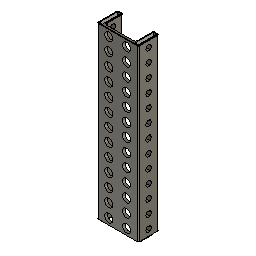
nxp_s32g3_support_plate (Autodesk Fusion 360 archive; units mm, degrees)
design "2u(ish) rail"
Autodesk Fusion 360 part; units mm, degrees
sketch "Sketch1" plane through (0, 0, 0) normal (0, 1, 0) x (1, 0, 0)
  line L0 (0, 0) -> (31.75, 0)
  line L1 (31.75, 0) -> (31.75, -130.8125)
  line L2 (31.75, -130.8125) -> (0, -130.8125)
  line L3 (0, -130.8125) -> (0, 0)
  line L4 (0, 0) -> (4.25, 0)
  line L5 (31.75, 0) -> (27.5, 0)
  line L6 (27.5, 0) -> (27.5, -130.8125)
  line L7 (4.25, 0) -> (4.25, -130.8125)
  circle A0 centre (9.0625, -5.0313) radius 3.1
  circle A1 centre (22.6875, -5.0313) radius 3.1
  circle A2 centre (9.0625, -15.0938) radius 3.1
  circle A3 centre (22.6875, -15.0938) radius 3.1
  circle A4 centre (9.0625, -25.1563) radius 3.1
  circle A5 centre (22.6875, -25.1563) radius 3.1
  circle A6 centre (9.0625, -35.2188) radius 3.1
  circle A7 centre (22.6875, -35.2188) radius 3.1
  circle A8 centre (9.0625, -45.2813) radius 3.1
  circle A9 centre (22.6875, -45.2813) radius 3.1
  circle A10 centre (9.0625, -55.3438) radius 3.1
  circle A11 centre (22.6875, -55.3438) radius 3.1
  circle A12 centre (9.0625, -65.4063) radius 3.1
  circle A13 centre (22.6875, -65.4063) radius 3.1
  circle A14 centre (9.0625, -75.4688) radius 3.1
  circle A15 centre (22.6875, -75.4688) radius 3.1
  circle A16 centre (9.0625, -85.5313) radius 3.1
  circle A17 centre (22.6875, -85.5313) radius 3.1
  circle A18 centre (9.0625, -95.5938) radius 3.1
  circle A19 centre (22.6875, -95.5938) radius 3.1
  circle A20 centre (9.0625, -105.6563) radius 3.1
  circle A21 centre (22.6875, -105.6563) radius 3.1
  circle A22 centre (9.0625, -115.7188) radius 3.1
  circle A23 centre (22.6875, -115.7188) radius 3.1
  circle A24 centre (9.0625, -125.7813) radius 3.1
  circle A25 centre (22.6875, -125.7813) radius 3.1
  dimension "d8" = 31.75
  dimension "d9" = 130.8125
  dimension "d11" = 4.25
  dimension "d12" = 4.25
  dimension "d15" = 6.2
  dimension "d16" = 5.0313
  dimension "d17" = 9.0625
  dimension "d18" = 6.2
  dimension "d19" = 5.0313
  dimension "d20" = 9.0625
  dimension "d23" = 10.0625
  dimension "d24" = 0
  constraint horizontal L0
  constraint vertical L1
  constraint horizontal L2
  constraint vertical L3
  constraint coincident L0.start L3.end
  constraint coincident L0 L4.end
  constraint perpendicular L1 L5
  constraint coincident L2 L6.end
  constraint perpendicular L2 L6
  constraint coincident L2 L7.end
  constraint perpendicular L2 L7
  measures "d8" distance of L0.start L0.end
  measures "d9" distance of L0.start L2.end
  measures "d11" distance of L0.start L4.end
  measures "d12" distance of L1 L6
  measures "d15" diameter of A0
  measures "d16" distance of L0 A0.centre
  measures "d17" distance of L3 A0.centre
  measures "d18" diameter of A1
  measures "d19" distance of L0 A1.centre
  measures "d20" distance of L1 A1.centre
extrude "Extrude1" add sketch "Sketch1" along normal blind 2 contours L0 L2 L6 L7 makes body 1
sketch "Sketch2" plane through (0, 0, 0) normal (0, 1, 0) x (1, 0, 0)
extrude "Extrude2" add sketch "Sketch1" along normal blind 15.875 contours L0 L2 L3 L4 L7 | L0 L1 L2 L5 L6 bodies 1
sketch "Sketch3" plane through (31.75, 0, 0) normal (1, 0, 0) x (0, 1, 0)
  line L0 (0, 130.8125) -> (0, 0)
  line L1 (0, 0) -> (15.875, 0)
  line L2 (15.875, 0) -> (15.875, 130.8125)
  line L3 (15.875, 130.8125) -> (0, 130.8125)
  circle A0 centre (7.9375, 5.0313) radius 2
  line L4 (0, 0) -> (0, 130.8125)
  line L5 (9.0922, 3.0313) -> (10.2469, 5.0313)
  line L6 (10.2469, 5.0313) -> (9.0922, 7.0313)
  line L7 (9.0922, 7.0313) -> (6.7828, 7.0313)
  line L8 (6.7828, 7.0313) -> (5.6281, 5.0313)
  line L9 (5.6281, 5.0313) -> (6.7828, 3.0313)
  line L10 (6.7828, 3.0313) -> (9.0922, 3.0313)
  line L11 (10.2469, 15.0938) -> (9.0922, 17.0938)
  line L12 (9.0922, 13.0938) -> (10.2469, 15.0938)
  line L13 (6.7828, 13.0938) -> (9.0922, 13.0938)
  line L14 (5.6281, 15.0938) -> (6.7828, 13.0938)
  line L15 (6.7828, 17.0938) -> (5.6281, 15.0938)
  line L16 (9.0922, 17.0938) -> (6.7828, 17.0938)
  line L17 (10.2469, 25.1563) -> (9.0922, 27.1563)
  line L18 (9.0922, 23.1563) -> (10.2469, 25.1563)
  line L19 (6.7828, 23.1563) -> (9.0922, 23.1563)
  line L20 (5.6281, 25.1563) -> (6.7828, 23.1563)
  line L21 (6.7828, 27.1563) -> (5.6281, 25.1563)
  line L22 (9.0922, 27.1563) -> (6.7828, 27.1563)
  line L23 (10.2469, 35.2188) -> (9.0922, 37.2188)
  line L24 (9.0922, 33.2188) -> (10.2469, 35.2188)
  line L25 (6.7828, 33.2188) -> (9.0922, 33.2188)
  line L26 (5.6281, 35.2188) -> (6.7828, 33.2188)
  line L27 (6.7828, 37.2188) -> (5.6281, 35.2188)
  line L28 (9.0922, 37.2188) -> (6.7828, 37.2188)
  line L29 (10.2469, 45.2813) -> (9.0922, 47.2813)
  line L30 (9.0922, 43.2813) -> (10.2469, 45.2813)
  line L31 (6.7828, 43.2813) -> (9.0922, 43.2813)
  line L32 (5.6281, 45.2813) -> (6.7828, 43.2813)
  line L33 (6.7828, 47.2813) -> (5.6281, 45.2813)
  line L34 (9.0922, 47.2813) -> (6.7828, 47.2813)
  line L35 (10.2469, 55.3438) -> (9.0922, 57.3438)
  line L36 (9.0922, 53.3438) -> (10.2469, 55.3438)
  line L37 (6.7828, 53.3438) -> (9.0922, 53.3438)
  line L38 (5.6281, 55.3438) -> (6.7828, 53.3438)
  line L39 (6.7828, 57.3438) -> (5.6281, 55.3438)
  line L40 (9.0922, 57.3438) -> (6.7828, 57.3438)
  line L41 (10.2469, 65.4063) -> (9.0922, 67.4063)
  line L42 (9.0922, 63.4063) -> (10.2469, 65.4063)
  line L43 (6.7828, 63.4063) -> (9.0922, 63.4063)
  line L44 (5.6281, 65.4063) -> (6.7828, 63.4063)
  line L45 (6.7828, 67.4063) -> (5.6281, 65.4063)
  line L46 (9.0922, 67.4063) -> (6.7828, 67.4063)
  line L47 (10.2469, 75.4688) -> (9.0922, 77.4688)
  line L48 (9.0922, 73.4688) -> (10.2469, 75.4688)
  line L49 (6.7828, 73.4688) -> (9.0922, 73.4688)
  line L50 (5.6281, 75.4688) -> (6.7828, 73.4688)
  line L51 (6.7828, 77.4688) -> (5.6281, 75.4688)
  line L52 (9.0922, 77.4688) -> (6.7828, 77.4688)
  line L53 (10.2469, 85.5313) -> (9.0922, 87.5313)
  line L54 (9.0922, 83.5313) -> (10.2469, 85.5313)
  line L55 (6.7828, 83.5313) -> (9.0922, 83.5313)
  line L56 (5.6281, 85.5313) -> (6.7828, 83.5313)
  line L57 (6.7828, 87.5313) -> (5.6281, 85.5313)
  line L58 (9.0922, 87.5313) -> (6.7828, 87.5313)
  line L59 (10.2469, 95.5938) -> (9.0922, 97.5938)
  line L60 (9.0922, 93.5938) -> (10.2469, 95.5938)
  line L61 (6.7828, 93.5938) -> (9.0922, 93.5938)
  line L62 (5.6281, 95.5938) -> (6.7828, 93.5938)
  line L63 (6.7828, 97.5938) -> (5.6281, 95.5938)
  line L64 (9.0922, 97.5938) -> (6.7828, 97.5938)
  line L65 (10.2469, 105.6563) -> (9.0922, 107.6563)
  line L66 (9.0922, 103.6563) -> (10.2469, 105.6563)
  line L67 (6.7828, 103.6563) -> (9.0922, 103.6563)
  line L68 (5.6281, 105.6563) -> (6.7828, 103.6563)
  line L69 (6.7828, 107.6563) -> (5.6281, 105.6563)
  line L70 (9.0922, 107.6563) -> (6.7828, 107.6563)
  line L71 (10.2469, 115.7188) -> (9.0922, 117.7188)
  line L72 (9.0922, 113.7188) -> (10.2469, 115.7188)
  line L73 (6.7828, 113.7188) -> (9.0922, 113.7188)
  line L74 (5.6281, 115.7188) -> (6.7828, 113.7188)
  line L75 (6.7828, 117.7188) -> (5.6281, 115.7188)
  line L76 (9.0922, 117.7188) -> (6.7828, 117.7188)
  line L77 (10.2469, 125.7813) -> (9.0922, 127.7813)
  line L78 (9.0922, 123.7813) -> (10.2469, 125.7813)
  line L79 (6.7828, 123.7813) -> (9.0922, 123.7813)
  line L80 (5.6281, 125.7813) -> (6.7828, 123.7813)
  line L81 (6.7828, 127.7813) -> (5.6281, 125.7813)
  line L82 (9.0922, 127.7813) -> (6.7828, 127.7813)
  point P0 (7.9375, 5.0313)
  dimension "d29" = 4
  dimension "d30" = 7.9375
  dimension "d31" = 5.0313
  dimension "d34" = 10.0625
  dimension "d35" = 0
  constraint coincident P0 A0.centre
  measures "d29" diameter of A0
  measures "d30" distance of P0 L4
  measures "d31" distance of L1 P0
extrude "Extrude3" cut sketch "Sketch3" against normal blind 65 contours A0 | A0 L5 L6 | A0 L6 L7 | A0 L5 L10 | A0 L7 L8 | A0 L9 L10 | A0 L8 L9 | L11 L12 L13 L14 L15 L16 | L17 L18 L19 L20 L21 L22 | L23 L24 L25 L26 L27 L28 | L29 L30 L31 L32 L33 L34 | L35 L36 L37 L38 L39 L40 | L41 L42 L43 L44 L45 L46 | L47 L48 L49 L50 L51 L52 | L53 L54 L55 L56 L57 L58 | L59 L60 L61 L62 L63 L64 | L65 L66 L67 L68 L69 L70 | L71 L72 L73 L74 L75 L76 | L77 L78 L79 L80 L81 L82 bodies 1
sketch "Sketch4" plane through (0, 0, 0) normal (0, 0, -1) x (1, 0, 0)
  line L0 (31.75, 0) -> (0, 0)
  line L1 (0, 0) -> (0, -15.875)
  line L2 (0, -15.875) -> (4.25, -15.875)
  line L3 (4.25, -15.875) -> (4.25, -2)
  line L4 (4.25, -2) -> (27.5, -2)
  line L5 (27.5, -2) -> (27.5, -15.875)
  line L6 (27.5, -15.875) -> (31.75, -15.875)
  line L7 (31.75, -15.875) -> (31.75, 0)
  line L8 (31.75, -15.875) -> (27.5, -15.875)
  line L9 (27.5, -15.875) -> (27.5, 0)
  line L10 (27.5, 0) -> (31.75, 0)
  line L11 (31.75, 0) -> (31.75, -15.875)
  line L12 (30.75, -14.875) -> (28.5, -14.875)
  line L13 (28.5, -14.875) -> (28.5, -1)
  line L14 (28.5, -1) -> (30.75, -1)
  line L15 (30.75, -1) -> (30.75, -14.875)
  line L16 (30.05, -1.7) -> (30.05, -14.175)
  line L17 (30.05, -14.175) -> (29.2, -14.175)
  line L18 (29.2, -14.175) -> (29.2, -1.7)
  line L19 (29.2, -1.7) -> (30.05, -1.7)
  line L20 (4.25, -15.875) -> (0, -15.875)
  line L21 (0, -15.875) -> (0, 0)
  line L22 (0, 0) -> (4.25, 0)
  line L23 (4.25, 0) -> (4.25, -15.875)
  line L24 (3.25, -1) -> (3.25, -14.875)
  line L25 (3.25, -14.875) -> (1, -14.875)
  line L26 (1, -14.875) -> (1, -1)
  line L27 (1, -1) -> (3.25, -1)
  line L28 (2.55, -1.7) -> (2.55, -14.175)
  line L29 (2.55, -14.175) -> (1.7, -14.175)
  line L30 (1.7, -14.175) -> (1.7, -1.7)
  line L31 (1.7, -1.7) -> (2.55, -1.7)
  line L32 (29.2, -3.7) -> (30.05, -3.7)
  line L33 (29.2, -12.175) -> (30.05, -12.175)
  line L34 (28.5, -12.875) -> (30.75, -12.875)
  line L35 (28.5, -3) -> (30.75, -3)
  line L36 (1.7, -3.7) -> (2.55, -3.7)
  line L37 (1.7, -12.175) -> (2.55, -12.175)
  line L38 (1, -12.875) -> (3.25, -12.875)
  line L39 (1, -3) -> (3.25, -3)
  dimension "d38" = 1
  dimension "d39" = 0.7
  dimension "d40" = 1
  dimension "d41" = 0.7
  dimension "d93" = 2
  dimension "d94" = 2
  dimension "d95" = 2
  dimension "d96" = 2
  dimension "d97" = 2
  dimension "d98" = 2
  dimension "d99" = 2
  dimension "d100" = 2
  constraint horizontal L8
  constraint vertical L9
  constraint horizontal L10
  constraint vertical L11
  constraint coincident L0 L9.end
  constraint coincident L6.end L7.start
  constraint horizontal L20
  constraint vertical L21
  constraint horizontal L22
  constraint vertical L23
  constraint coincident L0.end L1.start
  constraint coincident L2.end L3.start
  constraint coincident L18 L32.start
  constraint coincident L16 L32.end
  constraint perpendicular L16 L32
  constraint coincident L18 L33.start
  constraint coincident L16 L33.end
  constraint perpendicular L16 L33
  constraint coincident L13 L34.start
  constraint coincident L15 L34.end
  constraint perpendicular L15 L34
  constraint coincident L13 L35.start
  constraint coincident L15 L35.end
  constraint perpendicular L15 L35
  constraint coincident L30 L36.start
  constraint coincident L28 L36.end
  constraint perpendicular L28 L36
  constraint coincident L30 L37.start
  constraint coincident L28 L37.end
  constraint perpendicular L28 L37
  constraint coincident L24 L38.end
  constraint perpendicular L24 L38
  constraint coincident L26 L39.start
  constraint coincident L24 L39.end
  constraint perpendicular L24 L39
  measures "d93" distance of L19 L32
  measures "d94" distance of L17 L33
  measures "d95" distance of L12 L34
  measures "d96" distance of L14 L35
  measures "d97" distance of L31 L36
  measures "d98" distance of L29 L37
  measures "d99" distance of L25 L38
  measures "d100" distance of L27 L39
extrude "Extrude4" add sketch "Sketch4" along normal blind 2 separate body contours L16 L18 L32 L33 | L28 L30 L36 L37 makes body 2 at (29.2, 9.35, -0.6667) makes body 3 at (2.55, 6.525, -0.6667)
loft "Loft1" add profiles "Sketch4" section 1 face at (29.7667, 9.35, -2) section 2 contours L15 L16 L34 L35 | L13 L18 L34 L35 | L16 L18 L33 L34 | L16 L18 L32 L35 on bodies 2 bodies 1 3 2
loft "Loft2" add profiles "Sketch4" section 1 face at (2.2667, 9.35, -2) section 2 contours L24 L28 L38 L39 | L28 L30 L36 L39 | L26 L30 L38 L39 | L28 L30 L37 L38 on bodies 3 bodies 1 3
sketch "Sketch5" plane through (0, 0, 130.8125) normal (0, 0, 1) x (-1, 0, 0)
  line L0 (0, 0) -> (-31.75, 0)
  line L1 (-31.75, 0) -> (-31.75, -15.875)
  line L2 (-31.75, -15.875) -> (-27.5, -15.875)
  line L3 (-27.5, -15.875) -> (-27.5, -2)
  line L4 (-27.5, -2) -> (-4.25, -2)
  line L5 (-4.25, -2) -> (-4.25, -15.875)
  line L6 (-4.25, -15.875) -> (0, -15.875)
  line L7 (0, -15.875) -> (0, 0)
  line L8 (0, -15.875) -> (-4.25, -15.875)
  line L9 (-4.25, -15.875) -> (-4.25, 0)
  line L10 (-4.25, 0) -> (0, 0)
  line L11 (0, 0) -> (0, -15.875)
  line L12 (-27.5, -15.875) -> (-31.75, -15.875)
  line L13 (-31.75, -15.875) -> (-31.75, 0)
  line L14 (-31.75, 0) -> (-27.5, 0)
  line L15 (-27.5, 0) -> (-27.5, -15.875)
  line L16 (-0.9, -0.9) -> (-0.9, -14.975)
  line L17 (-0.9, -14.975) -> (-3.35, -14.975)
  line L18 (-3.35, -14.975) -> (-3.35, -0.9)
  line L19 (-3.35, -0.9) -> (-0.9, -0.9)
  line L20 (-2.7, -14.325) -> (-2.7, -1.55)
  line L21 (-2.7, -1.55) -> (-1.55, -1.55)
  line L22 (-1.55, -1.55) -> (-1.55, -14.325)
  line L23 (-1.55, -14.325) -> (-2.7, -14.325)
  line L24 (-30.85, -14.975) -> (-30.85, -0.9)
  line L25 (-30.85, -0.9) -> (-28.4, -0.9)
  line L26 (-28.4, -0.9) -> (-28.4, -14.975)
  line L27 (-28.4, -14.975) -> (-30.85, -14.975)
  line L28 (-29.05, -1.55) -> (-29.05, -14.325)
  line L29 (-29.05, -14.325) -> (-30.2, -14.325)
  line L30 (-30.2, -14.325) -> (-30.2, -1.55)
  line L31 (-30.2, -1.55) -> (-29.05, -1.55)
  dimension "d45" = 0.9
  dimension "d46" = 0.65
  dimension "d47" = 0.9
  dimension "d48" = 0.65
  constraint horizontal L8
  constraint vertical L9
  constraint horizontal L10
  constraint vertical L11
  constraint coincident L0 L9.end
  constraint coincident L6.end L7.start
  constraint horizontal L12
  constraint vertical L13
  constraint horizontal L14
  constraint vertical L15
  constraint coincident L0.end L1.start
  constraint coincident L2.end L3.start
extrude "Extrude5" cut sketch "Sketch5" against normal blind 2.5 contours L20 L21 L22 L23 | L28 L29 L30 L31 bodies 1
loft "Loft3" cut profiles "Sketch5" section 1 contours L16 L17 L18 L19 section 2 face at (2.3167, 5.8083, 128.3125) on bodies 1 bodies 1
loft "Loft4" cut profiles "Sketch5" section 1 contours L24 L25 L26 L27 section 2 face at (29.8167, 5.8083, 128.3125) on bodies 1 bodies 1
fillet "Fillet1" radius 0.25 4 edges at (1.225, 14.65, 129.5625) (3.025, 14.65, 129.5625) (1.225, 1.225, 129.5625) (3.025, 1.225, 129.5625) on bodies 1
fillet "Fillet2" radius 0.25 8 edges at (1.62, 14.255, 128.3125) (2.125, 14.325, 128.3125) (2.63, 14.255, 128.3125) (2.7, 7.9375, 128.3125) (2.63, 1.62, 128.3125) (2.125, 1.55, 128.3125) (1.62, 1.62, 128.3125) (1.55, 7.9375, 128.3125) on bodies 1
fillet "Fillet3" radius 0.25 4 edges at (28.725, 1.225, 129.5625) (30.525, 1.225, 129.5625) (28.725, 14.65, 129.5625) (30.525, 14.65, 129.5625) on bodies 1
fillet "Fillet4" radius 0.25 8 edges at (29.12, 14.255, 128.3125) (29.625, 14.325, 128.3125) (30.13, 14.255, 128.3125) (30.2, 7.9375, 128.3125) (30.13, 1.62, 128.3125) (29.625, 1.55, 128.3125) (29.12, 1.62, 128.3125) (29.05, 7.9375, 128.3125) on bodies 1
fillet "Fillet5" radius 1 6 edges at (31.75, 0, 65.4062) (31.75, 15.875, 65.4062) (27.5, 15.875, 65.4062) (4.25, 15.875, 65.4062) (0, 15.875, 65.4062) (0, 0, 65.4062) on bodies 1
fillet "Fillet6" radius 1.5 2 edges at (4.25, 2, 65.4062) (27.5, 2, 65.4062) on bodies 1
fillet "Fillet7" radius 0.25 16 edges at (0, 7.9375, 130.8125) (0.2929, 15.5821, 130.8125) (2.125, 15.875, 130.8125) (3.9571, 15.5821, 130.8125) (4.25, 9.1875, 130.8125) (4.6893, 2.4393, 130.8125) (15.875, 2, 130.8125) (27.0607, 2.4393, 130.8125) (27.5, 9.1875, 130.8125) (27.7929, 15.5821, 130.8125) (29.625, 15.875, 130.8125) (31.4571, 15.5821, 130.8125) (31.75, 7.9375, 130.8125) (31.4571, 0.2929, 130.8125) (15.875, 0, 130.8125) (0.2929, 0.2929, 130.8125) on bodies 1
fillet "Fillet8" radius 0.25 16 edges at (31.75, 7.9375, 0) (31.4571, 15.5821, 0) (29.625, 15.875, 0) (27.7929, 15.5821, 0) (27.5, 9.1875, 0) (27.0607, 2.4393, 0) (15.875, 2, 0) (4.6893, 2.4393, 0) (4.25, 9.1875, 0) (3.9571, 15.5821, 0) (2.125, 15.875, 0) (0.2929, 15.5821, 0) (0, 7.9375, 0) (0.2929, 0.2929, 0) (15.875, 0, 0) (31.4571, 0.2929, 0) on bodies 1
fillet "Fillet9" radius 0.25 8 edges at (30.4, 12.525, -1) (28.85, 12.525, -1) (30.4, 3.35, -1) (28.85, 3.35, -1) (2.9, 12.525, -1) (1.35, 12.525, -1) (2.9, 3.35, -1) (1.35, 3.35, -1) on bodies 1
fillet "Fillet10" radius 0.25 16 edges at (29.9824, 3.7676, -2) (29.625, 3.7, -2) (29.2676, 3.7676, -2) (29.2, 7.9375, -2) (29.2676, 12.1074, -2) (29.625, 12.175, -2) (29.9824, 12.1074, -2) (30.05, 7.9375, -2) (2.4824, 3.7676, -2) (2.125, 3.7, -2) (1.7676, 3.7676, -2) (1.7, 7.9375, -2) (1.7676, 12.1074, -2) (2.125, 12.175, -2) (2.4824, 12.1074, -2) (2.55, 7.9375, -2) on bodies 1
fillet "Fillet11" radius 0.25 16 edges at (1.0676, 12.8074, 0) (1, 7.9375, 0) (1.0676, 3.0676, 0) (2.125, 3, 0) (3.1824, 3.0676, 0) (3.25, 7.9375, 0) (3.1824, 12.8074, 0) (2.125, 12.875, 0) (28.5676, 12.8074, 0) (28.5, 7.9375, 0) (28.5676, 3.0676, 0) (29.625, 3, 0) (30.6824, 3.0676, 0) (30.75, 7.9375, 0) (30.6824, 12.8074, 0) (29.625, 12.875, 0) on bodies 1
equation "frame_width = 31.75 mm"
equation "frame_dist_base_screw = 5.0313 mm"
equation "frame_dist_scew_screw = 10.0625 mm"
equation "frame_heatinst_diameter = 4 mm"
equation "frame_align_top_offset_maj = 0.9 mm"
equation "frame_align_top_off_min = 0.65 mm"
equation "frame_4_height = 261.625 mm"
equation "d8 = frame_width"
equation "d9 = frame_4_height / 2"
equation "frame_side_offset = 4.25 mm"
equation "d11 = frame_side_offset"
equation "frame_thick_min = 2 mm"
equation "frame_dia_screw_struct = 6.2 mm"
equation "d15 = frame_dia_screw_struct"
equation "d16 = frame_dist_base_screw"
equation "d17 = frame_dist_scew_screw - 1 mm"
equation "d19 = frame_dist_base_screw"
equation "d20 = frame_dist_scew_screw - 1 mm"
equation "d23 = frame_dist_scew_screw"
equation "d25 = frame_thick_min"
equation "d27 = frame_width / 2"
equation "d29 = frame_heatinst_diameter"
equation "d30 = frame_width / 4"
equation "d31 = frame_dist_base_screw"
equation "d34 = frame_dist_scew_screw"
equation "frame_align_height = 3.05 mm"
equation "d45 = frame_align_top_offset_maj"
equation "d46 = frame_align_top_off_min"
equation "d47 = frame_align_top_offset_maj"
equation "d48 = frame_align_top_off_min"
equation "frame_4_height_Copy = 261.625 mm"
equation "frame_align_top_off_min_Copy = 0.65 mm"
equation "frame_dist_scew_screw_Copy = 10.0625 mm"
equation "frame_side_offset_Copy = 4.25 mm"
equation "frame_dist_base_screw_Copy = 5.0313 mm"
equation "frame_align_height_Copy = 3.05 mm"
equation "frame_heatinst_diameter_Copy = 2.1 mm"
equation "frame_thick_min_Copy = 2 mm"
equation "frame_align_top_offset_maj_Copy = 0.9 mm"
equation "frame_width_Copy = 31.75 mm"
equation "frame_dia_screw_struct_Copy = 6.2 mm"
equation "frame_4_height_Copy_1 = 261.625 mm"
equation "frame_align_top_off_min_Copy_1 = 0.65 mm"
equation "frame_dist_scew_screw_Copy_1 = 10.0625 mm"
equation "frame_side_offset_Copy_1 = 4.25 mm"
equation "frame_dist_base_screw_Copy_1 = 5.0313 mm"
equation "frame_align_height_Copy_1 = 3.05 mm"
equation "frame_heatinst_diameter_Copy_1 = 2.1 mm"
equation "frame_thick_min_Copy_1 = 2 mm"
equation "frame_align_top_offset_maj_Copy_1 = 0.9 mm"
equation "frame_width_Copy_1 = 31.75 mm"
equation "frame_dia_screw_struct_Copy_1 = 6.2 mm"
